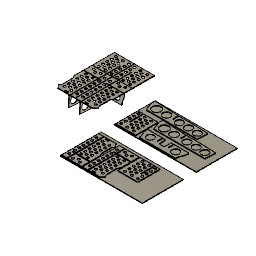
Element Platform 2026 EDITS v6 (Autodesk Fusion 360 design; units mm, degrees)
Autodesk Fusion 360 part; units mm, degrees
sketch "Sketch1" plane through (0, 0, 0) normal (0, 0, 1) x (1, 0, 0)
sketch "Sketch1 (2)" plane through (0, 0, 0) normal (0, 0, 1) x (1, 0, 0) in component "Vertical Legs"
  line L0 (1625.6, 355.6) -> (0, 355.6)
  line L1 (0, 355.6) -> (0, 0)
  line L2 (1600.2, 355.6) -> (1625.6, 0)
  line L3 (723.9, 196.85) -> (743.204, 196.85)
  line L4 (743.204, 196.85) -> (743.204, 38.1)
  line L5 (743.204, 38.1) -> (723.9, 38.1)
  line L6 (723.9, 38.1) -> (723.9, 196.85)
  line L7 (723.9, 38.1) -> (0, 0)
  spline S0 degree 5 poles (743.204, 38.1) (761.2257, 37.7534) (797.2365, 37.1233) (851.1553, 36.368) (922.849, 35.7465) (1012.1133, 35.6563) (1100.993, 36.3152) (1189.4556, 37.7859) (1277.4821, 40.1059) (1365.0877, 43.2452) (1452.3034, 47.1437) (1521.7892, 50.8208) (1573.7524, 53.8729) (1608.3285, 56.0362) (1625.6, 57.15) knots 0 0 0 0 0 0 0.1 0.2 0.3 0.4 0.5 0.6 0.7 0.8 0.9 1 1 1 1 1 1
  circle A0 centre (1449.6258, 201.2016) radius 107.95
  circle A1 centre (1184.2944, 195.7587) radius 107.95
  circle A2 centre (912.713, 197.466) radius 107.95
  circle A3 centre (230.1174, 183.7888) radius 127
  circle A4 centre (529.5022, 191.4938) radius 114.3
  line L8 (0, 102.1318) -> (86.8246, 355.6)
  point P0 (1194.054, 38.1)
  dimension "d18" = 1625.6
  dimension "d19" = 355.6
  dimension "d24" = 25.4
  dimension "d26" = 19.304
  dimension "d27" = 158.75
  dimension "d28" = 723.9
  dimension "d29" = 158.75
  dimension "d33" = 450.85
  dimension "d34" = 298.45
  dimension "d36" = 215.9
  dimension "d37" = 215.9
  dimension "d38" = 215.9
  dimension "d39" = 228.6
  dimension "d40" = 254
  constraint horizontal L0
  constraint vertical L1
  constraint coincident L0 L2.start
  constraint horizontal L3
  constraint vertical L4
  constraint vertical L6
  constraint coincident L1.end L7.end
  constraint horizontal L5
  constraint coincident L1 L8.start
  constraint coincident L0 L8.end
  measures "d18" distance of L1.end L2.end
  measures "d19" distance of L1.end L0.end
  measures "d24" distance of L0.start L2.start
  measures "d26" distance of L3.start L3.end
  measures "d27" distance of L3.start L5.end
  measures "d28" distance of L1 L6
  measures "d29" distance of L0 L3
  measures "d33" distance of L4.end P0
  measures "d34" distance of L0.start S0.end
  measures "d36" diameter of A0
  measures "d37" diameter of A1
  measures "d38" diameter of A2
  measures "d39" diameter of A4
  measures "d40" diameter of A3
sketch "Sketch1 (3)" plane through (0, 0, 0) normal (0, 0, 1) x (1, 0, 0) in component "Horizontal Piece"
  line L0 (0, 317.5) -> (0, 0) construction
  line L1 (460.502, 158.75) -> (441.198, 158.75)
  line L2 (441.198, 158.75) -> (441.198, 317.5)
  line L3 (441.198, 317.5) -> (460.502, 317.5)
  line L4 (460.502, 317.5) -> (460.502, 158.75)
  line L5 (460.502, 158.75) -> (441.198, 317.5) construction
  line L6 (441.198, 158.75) -> (460.502, 317.5) construction
  line L7 (615.8916, -79.3529) -> (615.8916, 317.5) construction
  circle A0 centre (241.3, 158.7502) radius 107.95
  spline S0 degree 5 poles (0.0945, 293.8725) (0.1549, 292.2355) (0.3196, 288.9985) (0.6975, 284.2574) (1.5745, 277.5639) (3.777, 266.1848) (7.5409, 249.6752) (12.8367, 229.161) (19.2578, 207.3532) (26.4381, 185.537) (33.9489, 164.7941) (41.389, 145.6307) (48.3923, 128.2736) (54.6722, 112.6705) (60.0502, 98.611) (64.4967, 85.7911) (68.0866, 73.8524) (70.9531, 62.4065) (73.2468, 51.0635) (75.0875, 39.459) (76.543, 27.2775) (77.4274, 16.8699) (77.9381, 8.6164) (78.2108, 2.9067) (78.3302, 0) knots 0 0 0 0 0 0 0.05 0.1 0.15 0.2 0.25 0.3 0.35 0.4 0.45 0.5 0.55 0.6 0.65 0.7 0.75 0.8 0.85 0.9 0.95 1 1 1 1 1 1
  line L8 (536.586, 139.7014) -> (536.586, 317.5)
  line L9 (76.8045, 37.1408) -> (79.8559, -37.1408)
  line L10 (-0.6192, 283.4968) -> (16.3074, 214.5018)
  arc A1 (536.586, 139.7014) -> (561.986, 114.3014) centre (561.986, 139.7014) ccw
  line L11 (78.3302, 0) -> (615.8916, 0)
  line L12 (615.8916, -10) -> (78.3302, -10)
  line L13 (78.3302, -10) -> (78.3302, 0)
  line L14 (561.986, 114.3014) -> (615.8916, 114.3014)
  line L15 (21.7951, 317.5) -> (536.586, 317.5)
  line L16 (3.1636, 302.6299) -> (12.1728, 313.0887)
  arc A2 (3.1636, 302.6299) -> (0.0945, 293.8725) centre (12.7858, 294.3412) ccw
  arc A3 (21.7951, 317.5) -> (12.1728, 313.0887) centre (21.7951, 304.8) ccw
  line L17 (615.8916, -10) -> (1153.4529, -10)
  line L18 (1153.4529, -10) -> (1153.4529, 0)
  line L19 (1153.4529, 0) -> (615.8916, 0)
  arc A4 (1231.6886, 293.8725) -> (1228.6195, 302.6299) centre (1218.9973, 294.3412) ccw
  line L20 (1228.6195, 302.6299) -> (1219.6103, 313.0887)
  arc A5 (1219.6103, 313.0887) -> (1209.988, 317.5) centre (1209.988, 304.8) ccw
  line L21 (695.1971, 139.7014) -> (695.1971, 317.5)
  arc A6 (669.7971, 114.3014) -> (695.1971, 139.7014) centre (669.7971, 139.7014) ccw
  line L22 (669.7971, 114.3014) -> (615.8916, 114.3014)
  line L23 (1209.988, 317.5) -> (695.1971, 317.5)
  spline S1 degree 5 poles (1231.6886, 293.8725) (1231.6282, 292.2355) (1231.4635, 288.9985) (1231.0856, 284.2574) (1230.2086, 277.5639) (1228.0061, 266.1848) (1224.2422, 249.6752) (1218.9464, 229.161) (1212.5253, 207.3532) (1205.345, 185.537) (1197.8342, 164.7941) (1190.3942, 145.6307) (1183.3908, 128.2736) (1177.1109, 112.6705) (1171.7329, 98.611) (1167.2864, 85.7911) (1163.6965, 73.8524) (1160.83, 62.4065) (1158.5363, 51.0635) (1156.6956, 39.459) (1155.2401, 27.2775) (1154.3558, 16.8699) (1153.845, 8.6164) (1153.5723, 2.9067) (1153.4529, 0) knots 0 0 0 0 0 0 0.05 0.1 0.15 0.2 0.25 0.3 0.35 0.4 0.45 0.5 0.55 0.6 0.65 0.7 0.75 0.8 0.85 0.9 0.95 1 1 1 1 1 1
  line L24 (-0.7612, 317.0361) -> (0.9501, 270.7088)
  line L25 (1232.5443, 317.0361) -> (1230.833, 270.7088)
  line L26 (1232.4023, 283.4968) -> (1215.4757, 214.5018)
  line L27 (1154.9786, 37.1408) -> (1151.9272, -37.1408)
  circle A7 centre (990.4831, 158.7502) radius 107.95
  line L28 (790.5851, 158.75) -> (790.5851, 317.5)
  line L29 (790.5851, 317.5) -> (771.2811, 317.5)
  line L30 (771.2811, 158.75) -> (790.5851, 158.75)
  line L31 (771.2811, 317.5) -> (771.2811, 158.75)
  point P0 (450.85, 238.125)
  point P1 (7.8441, 248.9993)
  point P2 (54.7294, 112.3366)
  point P3 (72.2296, 55.7615)
  point P4 (1231.7831, 0)
  point P5 (1223.939, 248.9993)
  point P6 (1177.0537, 112.3366)
  point P7 (1159.5535, 55.7615)
  dimension "d5_1" = 317.5
  dimension "d9_1" = 158.75
  dimension "d10_1" = 19.304
  dimension "d11_1" = 450.85
  dimension "d12_1" = 215.9
  dimension "d13_1" = 241.3
  dimension "d136_1" = 25.4
  dimension "d286" = 10
  dimension "d288" = 327.5
  dimension "d289" = 12.7
  dimension "d290" = 12.7
  dimension "d291" = 990.4831
  dimension "d292" = 158.7502
  dimension "d293" = 695.1971
  dimension "d294" = 54.7294
  dimension "d295" = 72.2296
  dimension "d296" = 76.216
  dimension "d297" = 55.7615
  dimension "d298" = 248.9993
  dimension "d299" = 214.5018
  dimension "d300" = 70.4861
  dimension "d301" = 79.3529
  constraint vertical L0
  constraint coincident L0.end origin
  constraint horizontal L1
  constraint perpendicular L1 L2
  constraint parallel L1 L3
  constraint parallel L2 L4
  constraint coincident L5 P0
  constraint coincident L6 P0
  constraint vertical L8
  constraint midpoint S0.end L9
  constraint symmetric L0.end L7 P4
  constraint midpoint P1 L10
  constraint tangent L8 A1
  constraint horizontal L11
  constraint horizontal L12
  constraint vertical L13
  constraint coincident L7 L14.end
  constraint tangent A1 L14
  constraint horizontal L14
  constraint coincident L7 L11.end
  constraint coincident L7 L12.start
  constraint tangent S0 A2
  constraint tangent L16 A2
  constraint tangent L15 A3
  constraint tangent L16 A3
  constraint midpoint S0.start L24
  constraint symmetric L1.start L7 L30.start
  constraint symmetric L1.end L7 L28.start
  constraint symmetric L2.end L7 L28.end
  constraint symmetric L3.end L7 L29.end
  constraint symmetric L7 A0 A7
  constraint symmetric L7 P1 P5
  constraint symmetric L7 P2 P6
  constraint symmetric L7 P3 P7
  constraint symmetric L7 S0.end L18.end
  constraint symmetric L7 L9.start L27.start
  constraint symmetric L7 L9.end L27.end
  constraint symmetric L7 L10.start L26.start
  constraint symmetric L7 L10.end L26.end
  constraint symmetric L7 L8.start L21.start
  constraint symmetric L7 A1.end A6.start
  constraint symmetric L7 A1 A6
  constraint symmetric L7 L12.end L17.end
  constraint symmetric L7 L14.end L22.end
  constraint symmetric L7 L11.end L19.end
  constraint symmetric L7 L12.start L17.start
  constraint symmetric L7 S0.start A4.start
  constraint symmetric L7 A2 A4
  constraint symmetric L7 L16.start A4.end
  constraint symmetric L7 L15.start A5.end
  constraint symmetric L7 L16.end L20.end
  constraint symmetric L7 A3 A5
  constraint symmetric L7 L24.start L25.start
  constraint symmetric L7 L24.end L25.end
  constraint horizontal L0.end L11.end
  constraint horizontal L0.start L3.end
  constraint horizontal L0.start L7.end
  measures "d5_1" distance of L0.end L0.start
  measures "d9_1" distance of L1.end L2.end
  measures "d10_1" distance of L2.end L3.end
  measures "d11_1" distance of L0 P0
  measures "d12_1" diameter of A0
  measures "d13_1" distance of L0 A0.centre
  measures "d136_1" radius of A1
  measures "d286" distance of S0.end L12.end
  measures "d288" distance of L12 L15
  measures "d289" radius of A2
  measures "d290" radius of A3
  measures "d291" distance of L0 A7.centre
  measures "d292" vertical distance of L0.end A7.centre
  measures "d293" distance of L0 L21
  measures "d294" distance of L0 P2
  measures "d295" distance of L0 P3
  measures "d296" angle of L10 L15
  measures "d297" distance of P3 L11
  measures "d298" distance of P1 L11
  measures "d299" distance of L10.end L11
  measures "d300" distance of P1 L13
  measures "d301" vertical distance of L0.end L7.start
extrude "Extrude1" add sketch "Sketch1 (2)" along normal blind 19.05 contours L0 L1 L2 L3 L4 L6 L7 S0 L8 makes body 1 in component "Vertical Legs"
extrude "Extrude2" add sketch "Sketch1 (3)" along normal blind 19.05 separate body contours L1 L2 L4 S0 L8 A1 L11 L14 L15 L16 A2 A3 L19 A4 L20 A5 L21 A6 L22 L23 S1 L28 L30 L31 | L9 L11 L12 L17 L19 L27 | L9 L12 L13 | L17 L18 L27 makes body 2 in component "Horizontal Piece"
extrude "Extrude1'" add sketch "Sketch1 (2)" along normal blind 19.05 separate body contours L0 L1 L2 L3 L4 L6 L7 S0 L8 makes body 3 in component "Vertical Piece 2"
move_body "Move9" bodies 1 to x (0, -1, 0) y (0, 0, 1) z (-1, 0, 0) at (760.016, 1021.8337, -261.8177) in component "Vertical Legs"
move_body "Move3" bodies 2 to x (1, 0, 0) y (0, 0, 1) z (0, -1, 0) at (0, 9.05, 29.05) in component "Horizontal Piece"
move_body "Move10" bodies 1 to x (1, 0, 0) y (0, 1, 0) z (0, 0, 1) at (30.5691, -288.8837, 252.7677) in component "Vertical Legs"
move_body "Move1" bodies 3 to x (0, -1, 0) y (0, 0, 1) z (-1, 0, 0) at (0, 0, 0) in component "Vertical Piece 2"
move_body "Move3'" bodies 3 to x (1, 0, 0) y (0, 1, 0) z (0, 0, 1) at (479.552, 732.95, -9.05) in component "Vertical Piece 2"
move_body "Move4" bodies 3 to x (1, 0, 0) y (0, 1, 0) z (0, 0, 1) at (-19.05, 0, 0) in component "Vertical Piece 2"
sketch "Sketch1 (4)" plane through (0, 0, 346.55) normal (0, 0, 1) x (1, 0, 0) in component "Top"
  line L0 (619.76, -846.455) -> (1210.31, -846.455)
  line L1 (1210.31, -846.455) -> (1210.31, 245.745)
  line L2 (1210.31, 245.745) -> (619.76, 245.745)
  line L3 (619.76, 245.745) -> (619.76, -846.455)
  spline S0 degree 5 poles (1143.5993, -846.455) (1143.2894, -844.852) (1142.7445, -841.7828) (1142.1516, -837.5896) (1141.8186, -832.7974) (1142.2227, -827.9765) (1143.5344, -824.0625) (1145.8635, -820.696) (1149.3352, -817.4241) (1154.0364, -813.7871) (1159.9612, -809.4042) (1166.9553, -804.0621) (1174.6606, -797.8004) (1182.5863, -790.8369) (1190.1767, -783.4973) (1196.8775, -776.1461) (1202.2063, -769.1149) (1205.8143, -762.638) (1207.5716, -756.7688) (1207.5844, -751.3575) (1206.0904, -746.1451) (1203.3879, -740.8241) (1199.7433, -735.1218) (1195.343, -728.8422) (1190.3163, -721.8449) (1184.7425, -714.0385) (1179.88, -707.103) (1176.0134, -701.5016) (1173.3384, -697.589) (1171.9766, -695.5881) knots 0 0 0 0 0 0 0.04 0.08 0.12 0.16 0.2 0.24 0.28 0.32 0.36 0.4 0.44 0.48 0.52 0.56 0.6 0.64 0.68 0.72 0.76 0.8 0.84 0.88 0.92 0.96 1 1 1 1 1 1
  spline S1 degree 5 poles (1167.5746, -681.2208) (1167.6097, -669.4496) (1167.68, -645.9073) (1167.7855, -610.5938) (1167.926, -563.5092) (1168.1018, -504.6535) (1168.2423, -457.5689) (1168.3478, -422.2554) (1168.4181, -398.7131) (1168.4532, -386.9419) knots 0 0 0 0 0 0 0.2 0.4 0.6 0.8 1 1 1 1 1 1
  spline S2 degree 5 poles (1168.4532, -386.9419) (1168.4612, -384.2575) (1168.6005, -379.0474) (1169.1791, -371.709) (1170.6655, -362.8442) (1173.5898, -353.1243) (1177.431, -344.5585) (1182.0411, -336.9413) (1187.2875, -330.0895) (1193.0578, -323.852) (1199.263, -318.115) (1204.5272, -313.8662) (1208.6296, -310.8539) (1211.432, -308.9219) (1212.85, -307.975) knots 0 0 0 0 0 0 0.1 0.2 0.3 0.4 0.5 0.6 0.7 0.8 0.9 1 1 1 1 1 1
  line L4 (1168.4235, -396.8842) -> (1168.4829, -376.9996)
  spline S3 degree 5 poles (1168.4532, 863.1919) (1168.4614, 860.4425) (1168.5982, 855.1193) (1169.1646, 847.6614) (1170.6252, 838.7145) (1173.5486, 828.9074) (1177.5018, 820.1831) (1182.4356, 812.319) (1188.3666, 805.3129) (1195.3031, 799.3574) (1202.9073, 794.1389) (1209.2041, 790.2288) (1213.8805, 787.2621) (1216.9549, 785.2438) (1218.4812, 784.2245) knots 0 0 0 0 0 0 0.1 0.2 0.3 0.4 0.5 0.6 0.7 0.8 0.9 1 1 1 1 1 1
  line L5 (1168.4235, 873.1342) -> (1168.4829, 853.2496)
  line L6 (1168.4235, 873.1342) -> (1168.4235, 898.525)
  line L7 (1168.4235, 873.1342) -> (1168.4532, 863.1919)
  circle A0 centre (876.9674, -69.9032) radius 34.925
  circle A1 centre (876.9674, -196.9032) radius 34.925
  circle A2 centre (876.9674, -450.9032) radius 34.925
  circle A3 centre (876.9674, -323.9032) radius 34.925
  circle A4 centre (876.9674, -704.9032) radius 34.925
  circle A5 centre (876.9674, -577.9032) radius 34.925
  circle A6 centre (978.5674, -641.4032) radius 34.925
  circle A7 centre (978.5674, -514.4032) radius 34.925
  circle A8 centre (978.5674, -387.4032) radius 34.925
  circle A9 centre (978.5674, -260.4032) radius 34.925
  circle A10 centre (978.5674, 101.5468) radius 34.925
  circle A11 centre (1080.1674, -704.9032) radius 34.925
  circle A12 centre (1080.1674, -577.9032) radius 34.925
  circle A13 centre (1080.1674, -450.9032) radius 34.925
  circle A14 centre (1080.1674, -323.9032) radius 34.925
  circle A15 centre (1080.1674, -196.9032) radius 34.925
  circle A16 centre (1080.1674, -69.9032) radius 34.925
  circle A17 centre (699.1674, -450.9032) radius 34.925
  circle A18 centre (699.1674, -704.9032) radius 34.925
  circle A19 centre (699.1674, -69.9032) radius 34.925
  circle A20 centre (699.1674, -196.9032) radius 34.925
  circle A21 centre (699.1674, -323.9032) radius 34.925
  circle A22 centre (699.1674, -577.9032) radius 34.925
  line L8 (955.675, -790.575) -> (874.395, -790.575)
  line L9 (874.395, -821.055) -> (955.675, -821.055)
  line L10 (965.835, -810.895) -> (965.835, -800.735)
  line L11 (965.835, -790.575) -> (864.235, -821.055) construction
  line L12 (864.235, -790.575) -> (965.835, -821.055) construction
  line L13 (864.235, -800.735) -> (864.235, -810.895)
  arc A23 (965.835, -800.735) -> (955.675, -790.575) centre (955.675, -800.735) ccw
  arc A24 (955.675, -821.055) -> (965.835, -810.895) centre (955.675, -810.895) ccw
  arc A25 (864.235, -810.895) -> (874.395, -821.055) centre (874.395, -810.895) ccw
  arc A26 (874.395, -790.575) -> (864.235, -800.735) centre (874.395, -800.735) ccw
  arc A27 (1167.5746, -681.2208) -> (1171.9766, -695.5881) centre (1192.9745, -681.2966) ccw
  circle A28 centre (699.1674, 101.5468) radius 34.925
  circle A29 centre (876.9674, 165.0468) radius 34.925
  circle A30 centre (978.5674, -133.4032) radius 34.925
  circle A31 centre (1080.1674, 165.0468) radius 34.925
  line L14 (1206.442, -312.2541) -> (1219.258, -303.6959)
  line L15 (1167.485, -711.2372) -> (1167.6642, -651.2043)
  line L16 (1168.3636, -416.9584) -> (1168.5428, -356.9255)
  line L17 (1149.2303, -875.5838) -> (1137.9683, -817.3262)
  line L18 (1187.4778, -718.3634) -> (1156.4754, -672.8129)
  line L19 (1212.0732, 788.5037) -> (1224.8892, 779.9454)
  line L20 (460.39, 742.98) -> (441.34, 742.98)
  line L21 (615.95, -749.7551) -> (615.95, 1226.0051) construction
  circle A32 centre (876.9674, 692.0968) radius 34.925
  circle A33 centre (978.5674, 628.5968) radius 34.925
  circle A34 centre (1080.1674, 692.0968) radius 34.925
  circle A35 centre (1080.1674, 565.0968) radius 34.925
  circle A36 centre (978.5674, 501.5968) radius 34.925
  circle A37 centre (876.9674, 565.0968) radius 34.925
  circle A38 centre (876.9674, 438.0968) radius 34.925
  circle A39 centre (1080.1674, 438.0968) radius 34.925
  circle A40 centre (699.1674, 438.0968) radius 34.925
  circle A41 centre (699.1674, 565.0968) radius 34.925
  circle A42 centre (699.1674, 692.0968) radius 34.925
  circle A43 centre (699.1674, 311.0968) radius 34.925
  circle A44 centre (876.9674, 311.0968) radius 34.925
  circle A45 centre (978.5674, 374.5968) radius 34.925
  circle A46 centre (1080.1674, 311.0968) radius 34.925
  circle A47 centre (1080.1674, 819.0968) radius 34.925
  circle A48 centre (876.9674, 819.0968) radius 34.925
  circle A49 centre (699.1674, 819.0968) radius 34.925
  circle A50 centre (978.5674, 755.5968) radius 34.925
  line L22 (1180.0362, 815.7281) -> (1188.7933, 804.8298)
  line L23 (619.76, 245.745) -> (1210.31, 245.745)
  line L24 (1210.31, 245.745) -> (1210.31, 906.145)
  line L25 (1210.31, 906.145) -> (619.76, 906.145)
  line L26 (619.76, 906.145) -> (619.76, 245.745)
  spline S4 degree 5 poles (64.3254, -681.2208) (64.2903, -669.4496) (64.22, -645.9073) (64.1145, -610.5938) (63.974, -563.5092) (63.7982, -504.6535) (63.6577, -457.5689) (63.5522, -422.2554) (63.4819, -398.7131) (63.4468, -386.9419) knots 0 0 0 0 0 0 0.2 0.4 0.6 0.8 1 1 1 1 1 1
  line L27 (64.415, -711.2372) -> (64.2358, -651.2043)
  line L28 (63.5364, -416.9584) -> (63.3572, -356.9255)
  circle A51 centre (354.9326, 438.0968) radius 34.925
  line L29 (21.59, -846.455) -> (21.59, 245.745)
  circle A52 centre (532.7326, 101.5468) radius 34.925
  line L30 (612.14, 245.745) -> (612.14, -846.455)
  spline S5 degree 5 poles (88.3007, -846.455) (88.6106, -844.852) (89.1555, -841.7828) (89.7484, -837.5896) (90.0814, -832.7974) (89.6773, -827.9765) (88.3656, -824.0625) (86.0365, -820.696) (82.5648, -817.4241) (77.8636, -813.7871) (71.9388, -809.4042) (64.9447, -804.0621) (57.2394, -797.8004) (49.3137, -790.8369) (41.7233, -783.4973) (35.0225, -776.1461) (29.6937, -769.1149) (26.0857, -762.638) (24.3284, -756.7688) (24.3156, -751.3575) (25.8096, -746.1451) (28.5121, -740.8241) (32.1567, -735.1218) (36.557, -728.8422) (41.5837, -721.8449) (47.1575, -714.0385) (52.02, -707.103) (55.8866, -701.5016) (58.5616, -697.589) (59.9234, -695.5881) knots 0 0 0 0 0 0 0.04 0.08 0.12 0.16 0.2 0.24 0.28 0.32 0.36 0.4 0.44 0.48 0.52 0.56 0.6 0.64 0.68 0.72 0.76 0.8 0.84 0.88 0.92 0.96 1 1 1 1 1 1
  line L31 (82.6697, -875.5838) -> (93.9317, -817.3262)
  line L32 (44.4222, -718.3634) -> (75.4246, -672.8129)
  circle A53 centre (253.3326, -260.4032) radius 34.925
  circle A54 centre (253.3326, -387.4032) radius 34.925
  spline S6 degree 5 poles (63.4468, -386.9419) (63.4388, -384.2575) (63.2995, -379.0474) (62.7209, -371.709) (61.2345, -362.8442) (58.3102, -353.1243) (54.469, -344.5585) (49.8589, -336.9413) (44.6125, -330.0895) (38.8422, -323.852) (32.637, -318.115) (27.3728, -313.8662) (23.2704, -310.8539) (20.468, -308.9219) (19.05, -307.975) knots 0 0 0 0 0 0 0.1 0.2 0.3 0.4 0.5 0.6 0.7 0.8 0.9 1 1 1 1 1 1
  line L33 (63.4765, -396.8842) -> (63.4171, -376.9996)
  line L34 (25.458, -312.2541) -> (12.642, -303.6959)
  circle A55 centre (253.3326, -514.4032) radius 34.925
  circle A56 centre (532.7326, 438.0968) radius 34.925
  circle A57 centre (151.7326, 165.0468) radius 34.925
  circle A58 centre (253.3326, 374.5968) radius 34.925
  circle A59 centre (354.9326, 165.0468) radius 34.925
  line L35 (21.59, 245.745) -> (612.14, 245.745)
  line L36 (612.14, 245.745) -> (21.59, 245.745)
  circle A60 centre (354.9326, 692.0968) radius 34.925
  line L37 (63.4765, 873.1342) -> (63.4468, 863.1919)
  line L38 (21.59, 906.145) -> (612.14, 906.145)
  circle A61 centre (354.9326, 819.0968) radius 34.925
  circle A62 centre (354.9326, -323.9032) radius 34.925
  circle A63 centre (354.9326, -704.9032) radius 34.925
  circle A64 centre (354.9326, -196.9032) radius 34.925
  circle A65 centre (151.7326, 311.0968) radius 34.925
  circle A66 centre (151.7326, -196.9032) radius 34.925
  circle A67 centre (532.7326, -577.9032) radius 34.925
  circle A68 centre (151.7326, -577.9032) radius 34.925
  circle A69 centre (151.7326, -450.9032) radius 34.925
  circle A70 centre (532.7326, -323.9032) radius 34.925
  circle A71 centre (354.9326, -450.9032) radius 34.925
  arc A72 (59.9234, -695.5881) -> (64.3254, -681.2208) centre (38.9255, -681.2966) ccw
  circle A73 centre (151.7326, -323.9032) radius 34.925
  circle A74 centre (532.7326, -450.9032) radius 34.925
  circle A75 centre (151.7326, 819.0968) radius 34.925
  circle A76 centre (151.7326, 692.0968) radius 34.925
  spline S7 degree 5 poles (63.4468, 863.1919) (63.4386, 860.4425) (63.3018, 855.1193) (62.7354, 847.6614) (61.2748, 838.7145) (58.3514, 828.9074) (54.3982, 820.1831) (49.4644, 812.319) (43.5334, 805.3129) (36.5969, 799.3574) (28.9927, 794.1389) (22.6959, 790.2288) (18.0195, 787.2621) (14.9451, 785.2438) (13.4188, 784.2245) knots 0 0 0 0 0 0 0.1 0.2 0.3 0.4 0.5 0.6 0.7 0.8 0.9 1 1 1 1 1 1
  line L39 (63.4765, 873.1342) -> (63.4171, 853.2496)
  line L40 (51.8638, 815.7281) -> (43.1067, 804.8298)
  line L41 (19.8268, 788.5037) -> (7.0108, 779.9454)
  circle A77 centre (532.7326, 692.0968) radius 34.925
  circle A78 centre (532.7326, 819.0968) radius 34.925
  line L42 (21.59, 245.745) -> (21.59, 906.145)
  circle A79 centre (532.7326, 565.0968) radius 34.925
  circle A80 centre (354.9326, 565.0968) radius 34.925
  circle A81 centre (151.7326, 565.0968) radius 34.925
  circle A82 centre (253.3326, 101.5468) radius 34.925
  circle A83 centre (151.7326, 438.0968) radius 34.925
  arc A84 (357.505, -821.055) -> (367.665, -810.895) centre (357.505, -810.895) ccw
  line L43 (367.665, -790.575) -> (266.065, -821.055) construction
  circle A85 centre (151.7326, -69.9032) radius 34.925
  line L44 (266.065, -790.575) -> (367.665, -821.055) construction
  circle A86 centre (532.7326, -69.9032) radius 34.925
  circle A87 centre (253.3326, 628.5968) radius 34.925
  circle A88 centre (253.3326, 755.5968) radius 34.925
  line L45 (63.4765, 873.1342) -> (63.4765, 898.525)
  circle A89 centre (354.9326, 311.0968) radius 34.925
  circle A90 centre (532.7326, 311.0968) radius 34.925
  circle A91 centre (253.3326, 501.5968) radius 34.925
  arc A92 (367.665, -800.735) -> (357.505, -790.575) centre (357.505, -800.735) ccw
  circle A93 centre (253.3326, -133.4032) radius 34.925
  circle A94 centre (354.9326, -577.9032) radius 34.925
  circle A95 centre (253.3326, -641.4032) radius 34.925
  circle A96 centre (532.7326, -704.9032) radius 34.925
  line L46 (276.225, -790.575) -> (357.505, -790.575)
  circle A97 centre (354.9326, -69.9032) radius 34.925
  line L47 (612.14, -846.455) -> (21.59, -846.455)
  line L48 (357.505, -821.055) -> (276.225, -821.055)
  arc A98 (266.065, -810.895) -> (276.225, -821.055) centre (276.225, -810.895) ccw
  circle A99 centre (151.7326, -704.9032) radius 34.925
  arc A100 (276.225, -790.575) -> (266.065, -800.735) centre (276.225, -800.735) ccw
  circle A101 centre (532.7326, -196.9032) radius 34.925
  line L49 (63.4765, -396.8842) -> (63.4171, -376.9996)
  line L50 (266.065, -810.895) -> (266.065, -800.735)
  line L51 (367.665, -800.735) -> (367.665, -810.895)
  line L52 (459.867, -868.52) -> (459.867, 644.8554)
  line L53 (434.467, 644.8554) -> (434.467, -868.52)
  line L54 (434.467, -868.52) -> (459.867, -868.52)
  line L55 (459.867, 644.8554) -> (434.467, 644.8554)
  line L56 (612.14, 906.145) -> (612.14, 245.745)
  line L57 (790.5851, -867.25) -> (790.5851, 646.1254)
  line L58 (790.5851, 646.1254) -> (771.5351, 646.1254)
  line L59 (771.5351, 646.1254) -> (771.5351, -867.25)
  line L60 (771.5351, -867.25) -> (790.5851, -867.25)
  point P0 (1143.7776, -824.2213)
  point P1 (1160.0795, -809.2779)
  point P2 (1204.2305, -765.127)
  point P3 (1204.2305, -742.7118)
  point P4 (1184.4147, -334.0289)
  point P5 (1184.4147, 810.2789)
  point P6 (915.035, -805.815)
  point P7 (615.95, 238.125)
  point P8 (47.4853, 810.2789)
  point P9 (615.95, -749.7551)
  point P10 (47.4853, -334.0289)
  point P11 (27.6695, -742.7118)
  point P12 (88.1224, -824.2213)
  point P13 (27.6695, -765.127)
  point P14 (316.865, -805.815)
  point P15 (615.95, 238.125)
  point P16 (622.3, -854.075)
  point P17 (622.3, -854.075)
  point P18 (71.8205, -809.2779)
  dimension "d54" = 590.55
  dimension "d55" = 1092.2
  dimension "d56" = 553.72
  dimension "d58" = 69.85
  dimension "d59" = 69.85
  dimension "d61" = 69.85
  dimension "d62" = 69.85
  dimension "d64" = 69.85
  dimension "d65" = 69.85
  dimension "d67" = 69.85
  dimension "d68" = 69.85
  dimension "d70" = 69.85
  dimension "d71" = 69.85
  dimension "d72" = 69.85
  dimension "d74" = 69.85
  dimension "d75" = 69.85
  dimension "d76" = 127
  dimension "d77" = 69.85
  dimension "d78" = 69.85
  dimension "d79" = 69.85
  dimension "d80" = 69.85
  dimension "d81" = 69.85
  dimension "d82" = 69.85
  dimension "d83" = 69.85
  dimension "d84" = 69.85
  dimension "d85" = 69.85
  dimension "d86" = 69.85
  dimension "d99" = 101.6
  dimension "d100" = 30.48
  dimension "d102" = 295.275
  dimension "d104" = 25.4
  dimension "d105" = 10.16
  dimension "d106" = 25.4
  dimension "d108" = 69.85
  dimension "d112" = 69.85
  dimension "d113" = 69.85
  dimension "d114" = 69.85
  dimension "d179" = 69.85
  dimension "d180" = 69.85
  dimension "d181" = 69.85
  dimension "d182" = 69.85
  dimension "d183" = 69.85
  dimension "d184" = 69.85
  dimension "d185" = 69.85
  dimension "d186" = 69.85
  dimension "d187" = 127
  dimension "d188" = 69.85
  dimension "d189" = 69.85
  dimension "d190" = 69.85
  dimension "d191" = 69.85
  dimension "d192" = 69.85
  dimension "d193" = 69.85
  dimension "d194" = 69.85
  dimension "d195" = 69.85
  dimension "d196" = 69.85
  dimension "d197" = 69.85
  dimension "d198" = 69.85
  dimension "d199" = 590.55
  dimension "d200" = 660.4
  constraint horizontal L0
  constraint vertical L1
  constraint horizontal L2
  constraint vertical L3
  constraint coincident L0 S0.start
  constraint midpoint S1.end L4
  constraint coincident S1 L4.start
  constraint midpoint S3.start L5
  constraint coincident L5.start L6.start
  constraint horizontal L8
  constraint parallel L8 L9
  constraint coincident L11 P6
  constraint coincident L12 P6
  constraint midpoint L12 P6
  constraint perpendicular L9 L13
  constraint coincident L11.start L8
  constraint coincident L11.start L10
  constraint tangent L8 A23
  constraint tangent L10 A23
  constraint coincident L12.end L9
  constraint coincident L12.end L10
  constraint tangent L9 A24
  constraint tangent L10 A24
  constraint equal A23 A24
  constraint coincident L11.end L13
  constraint coincident L11.end L9
  constraint tangent L13 A25
  constraint tangent L9 A25
  constraint equal A23 A25
  constraint coincident L12.start L13
  constraint coincident L12.start L8
  constraint tangent L13 A26
  constraint tangent L8 A26
  constraint equal A23 A26
  constraint tangent S1 A27
  constraint tangent S0 A27
  constraint midpoint S2.end L14
  constraint midpoint S1.start L15
  constraint midpoint S1.end L16
  constraint midpoint S0.start L17
  constraint midpoint S0.end L18
  constraint midpoint S3.end L19
  constraint midpoint P5 L22
  constraint horizontal L23
  constraint vertical L24
  constraint horizontal L25
  constraint vertical L26
  constraint symmetric L0.start L21 L30.end
  constraint symmetric L0.end L21 L29.start
  constraint symmetric L1.end L21 L29.end
  constraint symmetric L2.end L21 L30.start
  constraint symmetric S0.start L21 S5.start
  constraint symmetric P0 L21 P12
  constraint symmetric P1 L21 P18
  constraint symmetric P2 L21 P13
  constraint symmetric P3 L21 P11
  constraint symmetric S1.end L21 S4.end
  constraint symmetric P4 L21 P10
  constraint symmetric S2.end L21 S6.end
  constraint symmetric L4.start L21 L33.start
  constraint symmetric L4.end L21 L33.end
  constraint symmetric L5.end L21 L39.end
  constraint symmetric L5.start L21 L37.start
  constraint symmetric S3.start L21 L37.end
  constraint symmetric P5 L21 P8
  constraint symmetric S3.end L21 S7.end
  constraint symmetric L6.end L21 L45.end
  constraint symmetric A0 L21 A97
  constraint symmetric A1 L21 A64
  constraint symmetric A2 L21 A71
  constraint symmetric A3 L21 A62
  constraint symmetric A4 L21 A63
  constraint symmetric A5 L21 A94
  constraint symmetric A6 L21 A95
  constraint symmetric A7 L21 A55
  constraint symmetric A8 L21 A54
  constraint symmetric A9 L21 A53
  constraint symmetric A10 L21 A82
  constraint symmetric A11 L21 A99
  constraint symmetric A12 L21 A68
  constraint symmetric A13 L21 A69
  constraint symmetric A14 L21 A73
  constraint symmetric A15 L21 A66
  constraint symmetric A16 L21 A85
  constraint symmetric A17 L21 A74
  constraint symmetric A18 L21 A96
  constraint symmetric A19 L21 A86
  constraint symmetric A20 L21 A101
  constraint symmetric A21 L21 A70
  constraint symmetric A22 L21 A67
  constraint symmetric L11.start L21 L44.start
  constraint symmetric L12.start L21 L43.start
  constraint symmetric L11.end L21 L44.end
  constraint symmetric L12.end L21 L43.end
  constraint symmetric P6 L21 P14
  constraint symmetric L8.start L21 L46.start
  constraint symmetric L10.end L21 A100.end
  constraint symmetric A23 L21 A100
  constraint symmetric L9.end L21 L48.end
  constraint symmetric L10.start L21 A98.start
  constraint symmetric A24 L21 A98
  constraint symmetric L13.end L21 A84.end
  constraint symmetric L9.start L21 A84.start
  constraint symmetric A25 L21 A84
  constraint symmetric L13.start L21 A92.start
  constraint symmetric L8.end L21 A92.end
  constraint symmetric A26 L21 A92
  constraint symmetric S1.start L21 S4.start
  constraint symmetric S0.end L21 S5.end
  constraint symmetric A27 L21 A72
  constraint symmetric A28 L21 A52
  constraint symmetric A29 L21 A59
  constraint symmetric A30 L21 A93
  constraint symmetric A31 L21 A57
  constraint symmetric L14.start L21 L34.start
  constraint symmetric L14.end L21 L34.end
  constraint symmetric L15.start L21 L27.start
  constraint symmetric L15.end L21 L27.end
  constraint symmetric L16.start L21 L28.start
  constraint symmetric L16.end L21 L28.end
  constraint symmetric L17.start L21 L31.start
  constraint symmetric L17.end L21 L31.end
  constraint symmetric L18.start L21 L32.start
  constraint symmetric L18.end L21 L32.end
  constraint symmetric L19.start L21 L41.start
  constraint symmetric L19.end L21 L41.end
  constraint symmetric P9 L21 L21.start
  constraint symmetric L21 P15 P7
  constraint symmetric L21 A32 A60
  constraint symmetric L21 A33 A87
  constraint symmetric L21 A34 A76
  constraint symmetric L21 A35 A81
  constraint symmetric L21 A36 A91
  constraint symmetric L21 A37 A80
  constraint symmetric L21 A38 A51
  constraint symmetric L21 A39 A83
  constraint symmetric L21 A40 A56
  constraint symmetric L21 A41 A79
  constraint symmetric L21 A42 A77
  constraint symmetric L21 A43 A90
  constraint symmetric L21 A44 A89
  constraint symmetric L21 A45 A58
  constraint symmetric L21 A46 A65
  constraint symmetric L21 A47 A75
  constraint symmetric L21 A48 A61
  constraint symmetric L21 A49 A78
  constraint symmetric L21 A50 A88
  constraint symmetric L21 L22.start L40.start
  constraint symmetric L21 L22.end L40.end
  constraint symmetric L21 L1.end L29.end
  constraint symmetric L21 L24.end L38.start
  constraint coincident L30.start L36
  constraint symmetric L21 L26 L56
  measures "d54" distance of L0.start L0.end
  measures "d55" distance of L0.start L2.end
  measures "d56" distance of L2 S2.end
  measures "d58" diameter of A0
  measures "d59" diameter of A1
  measures "d61" diameter of A3
  measures "d62" diameter of A2
  measures "d64" diameter of A5
  measures "d65" diameter of A4
  measures "d67" diameter of A10
  measures "d68" diameter of A9
  measures "d70" diameter of A8
  measures "d71" diameter of A7
  measures "d72" diameter of A6
  measures "d74" diameter of A16
  measures "d75" diameter of A15
  measures "d76" distance of A16.centre A15.centre
  measures "d77" diameter of A14
  measures "d78" diameter of A13
  measures "d79" diameter of A12
  measures "d80" diameter of A11
  measures "d81" diameter of A19
  measures "d82" diameter of A20
  measures "d83" diameter of A21
  measures "d84" diameter of A17
  measures "d85" diameter of A22
  measures "d86" diameter of A18
  measures "d99" distance of L11.end L12.end
  measures "d100" distance of L12.start L11.end
  measures "d102" distance of L3 P6
  measures "d104" distance of L0 L9
  measures "d105" radius of A23
  measures "d106" radius of A27
  measures "d108" diameter of A28
  measures "d112" diameter of A29
  measures "d113" diameter of A30
  measures "d114" diameter of A31
  measures "d179" diameter of A32
  measures "d180" diameter of A37
  measures "d181" diameter of A38
  measures "d182" diameter of A44
  measures "d183" diameter of A36
  measures "d184" diameter of A45
  measures "d185" diameter of A34
  measures "d186" diameter of A35
  measures "d187" distance of A34.centre A35.centre
  measures "d188" diameter of A39
  measures "d189" diameter of A46
  measures "d190" diameter of A42
  measures "d191" diameter of A41
  measures "d192" diameter of A40
  measures "d193" diameter of A43
  measures "d194" diameter of A33
  measures "d195" diameter of A48
  measures "d196" diameter of A47
  measures "d197" diameter of A49
  measures "d198" diameter of A50
  measures "d199" distance of L2.end L1.end
  measures "d200" distance of L2.end L25.end
extrude "Extrude3" add sketch "Sketch1 (4)" along normal blind 19.05 separate body contours L0 L1 L2 S0 S1 S2 L4 L15 L16 L18 L23 L57 | L0 L2 L23 L57 L59 | A27 L15 L18 | L0 L2 L3 L23 L59 makes body 4 in component "Top"
extrude "Extrude1''" add sketch "Sketch1 (4)" along normal blind 19.05 separate body contours S4 L27 L28 L29 S5 L32 S6 L33 L35 L36 L47 L49 L53 | L27 L32 A72 | L35 L36 L47 L52 L53 | L30 L35 L36 L47 L52 makes body 5 in component "TOP 2"
extrude "Extrude1'''" add sketch "Sketch1 (4)" along normal blind 19.05 separate body contours L35 L36 L52 L53 L55 | L35 L36 L38 L42 L52 L53 L55 L56 makes body 6 in component "TOP 3"
extrude "Extrude1''''" add sketch "Sketch1 (4)" along normal blind 19.05 separate body contours L2 L23 L24 L25 L26 L57 L58 L59 | L2 L23 L57 L58 L59 makes body 7 in component "TOP 4"
sketch "Sketch3" plane through (0, 0, 346.55) normal (0, 0, 1) x (-1, 0, 0) in component "Top"
  line L0 (-441.198, -9.05) -> (-21.7951, -9.05)
  line L1 (-21.7951, -9.05) -> (-21.7951, 10)
  line L2 (-21.7951, 10) -> (-441.198, 10)
  line L3 (-441.198, 10) -> (-441.198, -9.05)
  line L4 (-460.502, 867.25) -> (-460.502, -646.1254)
  line L5 (-441.452, -646.1254) -> (-441.452, 867.25)
  line L6 (-441.452, 867.25) -> (-460.502, 867.25)
  line L7 (-790.5851, 867.25) -> (-790.5851, -646.1254)
  line L8 (-771.5351, -646.1254) -> (-771.5351, 867.25)
  line L9 (-771.5351, 867.25) -> (-790.5851, 867.25)
  line L10 (-1209.988, -9.05) -> (-790.5851, -9.05)
  line L11 (-790.5851, -9.05) -> (-790.5851, 10)
  line L12 (-790.5851, 10) -> (-1209.988, 10)
  line L13 (-1209.988, 10) -> (-1209.988, -9.05)
  line L14 (-536.586, -9.05) -> (-460.502, -9.05)
  line L15 (-460.502, -9.05) -> (-460.502, 10)
  line L16 (-460.502, 10) -> (-536.586, 10)
  line L17 (-771.2811, -9.05) -> (-695.1971, -9.05)
  line L18 (-695.1971, 10) -> (-771.2811, 10)
  line L19 (-771.2811, 10) -> (-771.2811, -9.05)
  line L20 (-1209.988, -9.05) -> (-1219.6103, -9.05)
  line L21 (-1209.988, -9.05) -> (-1209.988, 10)
  line L22 (-1209.988, 10) -> (-1219.6103, 10)
  line L23 (-1219.6103, 10) -> (-1219.6103, -9.05)
  line L24 (-12.1728, -9.05) -> (-21.7951, -9.05)
  line L25 (-12.1728, -9.05) -> (-12.1728, 10)
  line L26 (-12.1728, 10) -> (-21.7951, 10)
  line L27 (-21.7951, 10) -> (-21.7951, -9.05)
  line L28 (-1228.6195, -9.05) -> (-1219.6103, -9.05)
  line L29 (-1219.6103, -9.05) -> (-1219.6103, 10)
  line L30 (-1219.6103, 10) -> (-1228.6195, 10)
  line L31 (-1228.6195, 10) -> (-1228.6195, -9.05)
  line L32 (-12.1728, -9.05) -> (-3.1636, -9.05)
  line L33 (-3.1636, -9.05) -> (-3.1636, 10)
  line L34 (-3.1636, 10) -> (-12.1728, 10)
  line L35 (-12.1728, 10) -> (-12.1728, -9.05)
  line L36 (-771.2811, -9.05) -> (-771.5351, -9.05)
  line L37 (-771.5351, -9.05) -> (-771.5351, 12.3079)
  line L38 (-771.5351, 12.3079) -> (-771.2811, 12.3079)
  line L39 (-771.2811, 12.3079) -> (-771.2811, -9.05)
  line L40 (-441.198, 10) -> (-441.452, 10)
  line L41 (-441.452, 10) -> (-441.452, -10.0217)
  line L42 (-441.452, -10.0217) -> (-441.198, -10.0217)
  line L43 (-441.198, -10.0217) -> (-441.198, 10)
  line L44 (-790.5851, -646.1254) -> (-771.5351, -646.1254)
  line L45 (-460.502, -646.1254) -> (-441.452, -646.1254)
  line L46 (-536.586, 10) -> (-536.586, -9.05)
  line L47 (-695.1971, -9.05) -> (-695.1971, 10)
  constraint horizontal L36
  constraint vertical L37
  constraint horizontal L38
  constraint vertical L39
  constraint coincident L8 L37.end
  constraint coincident L17.start L19.end
  constraint horizontal L40
  constraint vertical L41
  constraint horizontal L42
  constraint vertical L43
  constraint coincident L5 L41.end
  constraint coincident L2.end L3.start
extrude "Extrude7" cut sketch "Sketch3" along normal blind 6.35 bodies 4 in component "Top"
extrude "Extrude2'" cut sketch "Sketch3" along normal blind 6.35 bodies 5 in component "TOP 2"
extrude "Extrude2''" cut sketch "Sketch3" along normal blind 6.35 bodies 6 in component "TOP 3"
extrude "Extrude2'''" cut sketch "Sketch3" along normal blind 6.35 bodies 7 in component "TOP 4"
sketch "Sketch1 (5)" plane through (0, 0, 0) normal (0, 0, 1) x (1, 0, 0) in component "Plywood"
  line L0 (1524, -609.6) -> (3962.4, -609.6)
  line L1 (3962.4, -609.6) -> (3962.4, 609.6)
  line L2 (3962.4, 609.6) -> (1524, 609.6)
  line L3 (1524, 609.6) -> (1524, -609.6)
  line L4 (1524, -990.6) -> (3962.4, -990.6)
  line L5 (3962.4, -990.6) -> (3962.4, -2209.8)
  line L6 (3962.4, -2209.8) -> (1524, -2209.8)
  line L7 (1524, -2209.8) -> (1524, -990.6)
  dimension "d201" = 2438.4
  dimension "d202" = 1219.2
  dimension "d203" = 1524
  dimension "d205" = 609.6
  dimension "d282" = 2438.4
  dimension "d283" = 1219.2
  dimension "d284" = 1524
  dimension "d285" = 381
  constraint horizontal L0
  constraint vertical L1
  constraint horizontal L2
  constraint vertical L3
  constraint horizontal L4
  constraint vertical L5
  constraint horizontal L6
  constraint vertical L7
  measures "d201" distance of L0.start L0.end
  measures "d202" distance of L0.start L2.end
  measures "d203" distance of origin L3
  measures "d205" vertical distance of origin L2.end
  measures "d282" distance of L4.start L4.end
  measures "d283" distance of L4.start L6.end
  measures "d284" distance of origin L7
  measures "d285" distance of L0 L4
extrude "Extrude1'''''" add sketch "Sketch1 (5)" along normal blind 19.05 separate body makes body 8 at (2336.8, 203.2, 0) makes body 9 at (2336.8, -1397, 0) in component "Plywood"
other "Arrange1"
component "Vertical Legs" placed x (1, 0, 0) y (0, 1, 0) z (0, 0, 1) at (0, 0, 0)
component "Vertical Piece 2" placed x (1, 0, 0) y (0, 1, 0) z (0, 0, 1) at (0, 0, 0)
component "Horizontal Piece" placed x (1, 0, 0) y (0, 1, 0) z (0, 0, 1) at (0, 0, 0)
component "Top" placed x (1, 0, 0) y (0, 1, 0) z (0, 0, 1) at (0, 0, -6.35)
component "TOP 2" placed x (1, 0, 0) y (0, 1, 0) z (0, 0, 1) at (0, 0, -6.35)
component "TOP 3" placed x (1, 0, 0) y (0, 1, 0) z (0, 0, 1) at (0, 0, -6.35)
component "TOP 4" placed x (1, 0, 0) y (0, 1, 0) z (0, 0, 1) at (0, 0, -6.35)
component "CNC" placed x (1, 0, 0) y (0, 1, 0) z (0, 0, 1) at (0, 0, 0)
component "Arrange1" placed x (1, 0, 0) y (0, 1, 0) z (0, 0, 1) at (0, 0, 0)
component "Plywood" placed x (1, 0, 0) y (0, 1, 0) z (0, 0, 1) at (0, 0, 0) in component "CNC"
component "Envelope1(Qty: 1)" placed x (1, 0, 0) y (0, 1, 0) z (0, 0, 1) at (1524, -2209.8, 19.05) in component "Arrange1"
component "Envelope2(Qty: 1)" placed x (1, 0, 0) y (0, 1, 0) z (0, 0, 1) at (1524, -609.6, 19.05) in component "Arrange1"
component "Top" placed x (1, 0, 0) y (0, -1, 0) z (0, 0, -1) at (-594.3599, 271.145, 365.6) in component "Envelope1(Qty: 1)"
component "TOP 2" placed x (-1, 0, 0) y (0, 1, 0) z (0, 0, -1) at (1253.4153, 871.855, 365.6) in component "Envelope1(Qty: 1)"
component "TOP 3" placed x (1, 0, 0) y (0, -1, 0) z (0, 0, -1) at (1235.6376, 1363.345, 365.6) in component "Envelope1(Qty: 1)"
component "Vertical Legs" placed x (0, 0, 1) y (-1, 0, 0) z (0, -1, 0) at (758.35, 1183.378, -771.5351) in component "Envelope2(Qty: 1)"
component "Horizontal Piece" placed x (1, 0, 0) y (0, 0, -1) z (0, 1, 0) at (643.0235, 6.35, 9.05) in component "Envelope2(Qty: 1)"
component "Vertical Piece 2" placed x (0, 0, 1) y (-1, 0, 0) z (0, -1, 0) at (1368.1703, 801.006, -441.452) in component "Envelope2(Qty: 1)"
component "TOP 4" placed x (1, 0, 0) y (0, -1, 0) z (0, 0, -1) at (-594.3599, 931.5451, 365.6) in component "Envelope2(Qty: 1)"
equation "PLYWOOD = 0.75 in" comment "change as needed"
equation "Tolerance = 0.01 in" comment "+.1-.25mm"
equation "d18 = 35.5 in + 28.5 in"
equation "d26 = Tolerance + PLYWOOD"
equation "d33 = ( 35.5 / 2 ) * 1 in"
equation "d41 = PLYWOOD"
equation "d54 = 23.75 in - 0.5 in"
equation "d102 = ( 23.25 / 2 ) * 1 in"
equation "d9 = ( 12.5 / 2 ) * 1 in"
equation "d10 = Tolerance"
equation "d9_1 = ( 12.5 / 2 ) * 1 in"
equation "d10_1 = Tolerance + PLYWOOD"
equation "d47_1 = PLYWOOD"
equation "d165 = PLYWOOD"
equation "d206 = PLYWOOD"
equation "d238 = PLYWOOD"
equation "d240 = PLYWOOD"
equation "d242 = PLYWOOD"
equation "d244 = PLYWOOD"
equation "d327 = -PLYWOOD"
